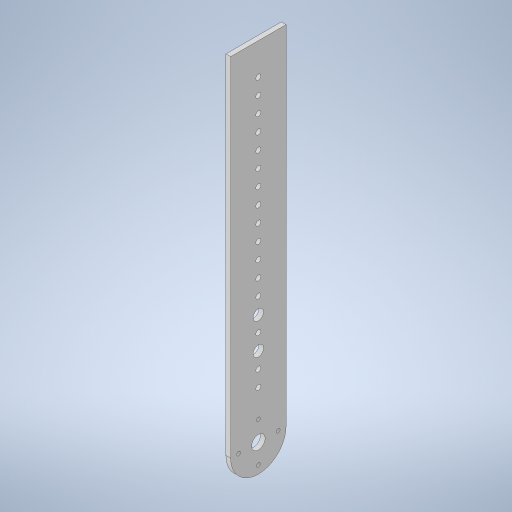
# Autodesk Inventor part: shoulder2_upper_plate
Saved by Autodesk Inventor 2024 (Build 280153000, 153)
## iProperties
Created: 2025-08-05
Part Number: shoulder2_upper_plate
Material: 一般
Document SubType Name: Modeling
Designer: HosodaLab2
Density: 1 g/cm^3
Appearance: 既定
Author: HosodaLab2
Autodesk Inventor part; units mm, degrees
ref_plane "YZ Plane" through (0, 0, 0) normal (1, 0, 0) x (0, 1, 0)
ref_plane "XZ Plane" through (0, 0, 0) normal (0, 1, 0) x (-1, 0, 0)
ref_plane "XY Plane" through (0, 0, 0) normal (0, 0, 1) x (1, 0, 0)
sketch "スケッチ1" plane through (0, 0, 0) normal (0, 1, 0) x (-1, 0, 0)
  line L0 (0, 0) -> (-35, 0)
  line L1 (-35, 0) -> (-35, -220)
  line L2 (-35, -220) -> (0, -220)
  line L3 (0, -220) -> (0, 0)
  arc A0 (-35, -220) -> (0, -220) centre (-17.5, -220) ccw
  dimension "d0" = 35
  dimension "d1" = 220
  dimension "d2" = 17.5
  constraints: 8 end point, 2 parallel, 2 point on circle, 1 centre point, 1 horizontal, 1 perpendicular
  measures "d0" distance of L2.end L1.end
  measures "d1" distance of L1.end L0.end
  measures "d2" radius of A0
extrude "押し出し1" add sketch "スケッチ1" along normal blind 3
sketch "スケッチ2" plane through (0, 3, 0) normal (0, 1, 0) x (1, 0, 0)
  line L0 (0, 0) -> (35, 0) construction
  line L1 (17.5, 0) -> (17.5, 237.5) construction
  arc A0 (35, 220) -> (0, 220) centre (17.5, 220) ccw construction
  constraints: 2 end point, 1 coincident, 1 midpoint, 1 point on circle, 1 vertical
hole "穴1" at (17.5, 3, -220) direction (0, -1, 0) diameter 8.5 end through all
sketch "スケッチ3" plane through (0, 3, 0) normal (0, 1, 0) x (1, 0, 0)
  circle A0 centre (17.5, 220) radius 4.25 projected
  circle A1 centre (17.5, 220) radius 12.5
  point P0 (0, 0)
  point P1 (5, 220)
  point P2 (30, 220)
  point P3 (17.5, 232.5)
  point P4 (17.5, 207.5)
  dimension "d12" = 25
  constraints: 4 point on circle, 1 centre point, 1 coincident
  measures "d12" diameter of A1
hole "穴2" at (5, 3, -220) at (30, 3, -220) at (17.5, 3, -232.5) at (17.5, 3, -207.5) direction (0, -1, 0) diameter 2.459 end through all thread size "M3x0.5" class "6H" standard "ISO Metric profile"
sketch "スケッチ4" plane through (0, 3, 0) normal (0, 1, 0) x (1, 0, 0)
  line L0 (0, 0) -> (35, 0) construction
  line L1 (17.5, 0) -> (17.5, 237.5) construction
  arc A0 (35, 220) -> (0, 220) centre (17.5, 220) ccw construction
  point P0 (17.5, 190)
  point P1 (17.5, 180)
  point P2 (17.5, 170)
  point P3 (17.5, 160)
  point P4 (17.5, 150)
  point P5 (17.5, 140)
  point P6 (17.5, 130)
  point P7 (17.5, 120)
  point P8 (17.5, 110)
  point P9 (17.5, 100)
  point P10 (17.5, 90)
  point P11 (17.5, 80)
  point P12 (17.5, 70)
  point P13 (17.5, 60)
  point P14 (17.5, 50)
  point P15 (17.5, 40)
  point P16 (17.5, 30)
  point P17 (17.5, 20)
  point P18 (17.5, 10)
  dimension "d22" = 10
  dimension "d27" = 30
  constraints: 2 end point, 2 vertical, 1 midpoint, 1 point on circle, 1 point on line, 18 other
  measures "d22" distance of point (17.5, 190) point (17.5, 180)
  measures "d27" distance of A0.centre point (17.5, 190)
hole "穴3" at (17.5, 3, -190) at (17.5, 3, -180) at (17.5, 3, -170) at (17.5, 3, -160) at (17.5, 3, -150) at (17.5, 3, -140) at (17.5, 3, -130) at (17.5, 3, -120) at (17.5, 3, -110) at (17.5, 3, -100) at (17.5, 3, -90) at (17.5, 3, -80) at (17.5, 3, -70) at (17.5, 3, -60) at (17.5, 3, -50) at (17.5, 3, -40) at (17.5, 3, -30) at (17.5, 3, -20) direction (0, -1, 0) diameter 3.2 end through all
sketch "スケッチ5" plane through (0, 3, 0) normal (0, 1, 0) x (1, 0, 0)
  circle A0 centre (17.5, 160) radius 1.6 projected
  circle A1 centre (17.5, 170) radius 1.6 projected
  point P0 (0, 0)
  point P1 (17.5, 150.1909)
  constraints: 1 coincident
hole "穴4" at (17.5, 3, -150.1909) at (17.5, 3, -170) direction (0, -1, 0) diameter 6.6 end through all
